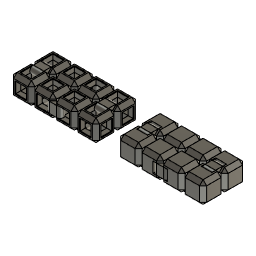
cubes v4 (Autodesk Fusion 360 design; units mm, degrees)
Autodesk Fusion 360 part; units mm, degrees
note: some values were not read from the file. Chosen so that the rebuilt part matches the saved one: which bodies a step acts on; which face or edge a step refers to. Set by a fixed rule: which sketch regions a step uses.
(part 1 of 2)
sketch "Sketch1" plane through (0, 0, 0) normal (0, 0, 1) x (1, 0, 0) in component "Cube"
  line L0 (0, 0) -> (50, 0)
  line L1 (50, 0) -> (50, -50)
  line L2 (50, -50) -> (0, -50)
  line L3 (0, -50) -> (0, 0)
  line L4 (50.2, 0) -> (100.2, 0)
  line L5 (100.2, 0) -> (100.2, -50)
  line L6 (100.2, -50) -> (50.2, -50)
  line L7 (50.2, -50) -> (50.2, 0)
  dimension "d1" = 50
  dimension "d2" = 50
  dimension "d3" = 50
  dimension "d4" = 50
  dimension "d5" = 0.2
  constraint horizontal L0
  constraint vertical L1
  constraint horizontal L2
  constraint vertical L3
  constraint coincident L0.start L3.end
  constraint horizontal L4
  constraint vertical L5
  constraint horizontal L6
  constraint vertical L7
  constraint collinear L0 L4
  measures "d1" distance of L1.end L2.end
  measures "d2" distance of L0.end L1.end
  measures "d3" distance of L4.start L4.end
  measures "d4" distance of L4.start L6.end
  measures "d5" distance of L1 L7
extrude "Extrude1" add sketch "Sketch1" along normal blind 50 makes body 1 at (16.6667, 0, 16.6667) makes body 2 at (100.2, -16.6667, 16.6667) in component "Cube"
sketch "Sketch2" plane through (0, 0, 0) normal (0, 0, -1) x (1, 0, 0) in component "Cube"
  line L0 (50, 50) -> (0, 50)
  line L1 (0, 50) -> (0, 0)
  line L2 (0, 0) -> (50, 0)
  line L3 (50, 0) -> (50, 50)
  line L4 (50, 12.5) -> (33.2333, 12.5)
  line L5 (33.2333, 12.5) -> (33.2333, 37.5)
  line L6 (33.2333, 37.5) -> (50, 37.5)
  line L7 (50, 37.5) -> (50, 12.5)
  line L8 (50.1, 12.7) -> (33.4333, 12.7)
  line L9 (33.4333, 12.7) -> (33.4333, 37.3)
  line L10 (33.4333, 37.3) -> (50.1, 37.3)
  line L11 (50.1, 37.3) -> (50.1, 12.7)
  line L12 (0, 25) -> (50, 25) construction
  dimension "d8" = 0.1
  dimension "d9" = 0.2
  dimension "d10" = 0.2
  dimension "d11" = 0.2
  dimension "d12" = 25
  dimension "d13" = 16.7667
  constraint horizontal L4
  constraint vertical L5
  constraint horizontal L6
  constraint vertical L7
  constraint coincident L3 L4.start
  constraint horizontal L8
  constraint vertical L9
  constraint horizontal L10
  constraint vertical L11
  constraint midpoint L1 L12.start
  constraint midpoint L3 L12.end
  constraint symmetric L4 L6 L12
  measures "d8" distance of L7 L11
  measures "d9" distance of L4 L8
  measures "d10" distance of L6 L10
  measures "d11" distance of L5 L9
  measures "d12" distance of L4.end L5.end
  measures "d13" distance of L4.start L4.end
sketch "Sketch3" plane through (0, 0, 0) normal (0, 0, -1) x (1, 0, 0) in component "Cube"
  line L0 (100.2, 50) -> (50.2, 50)
  line L1 (50.2, 50) -> (50.2, 0)
  line L2 (50.2, 0) -> (100.2, 0)
  line L3 (100.2, 0) -> (100.2, 50)
  line L4 (100.2, 25) -> (50.2, 25) construction
  line L5 (66.9667, 12.5) -> (50.2, 12.5)
  line L6 (50.2, 12.5) -> (50.2, 37.5)
  line L7 (50.2, 37.5) -> (66.9667, 37.5)
  line L8 (66.9667, 37.5) -> (66.9667, 12.5)
  line L9 (66.7667, 12.7) -> (50.1, 12.7)
  line L10 (50.1, 12.7) -> (50.1, 37.3)
  line L11 (50.1, 37.3) -> (66.7667, 37.3)
  line L12 (66.7667, 37.3) -> (66.7667, 12.7)
  dimension "d19" = 0.2
  dimension "d20" = 0.2
  dimension "d21" = 0.2
  dimension "d22" = 25
  dimension "d23" = 0.1
  dimension "d24" = 16.7667
  constraint midpoint L3 L4.start
  constraint midpoint L1 L4.end
  constraint horizontal L5
  constraint vertical L6
  constraint horizontal L7
  constraint vertical L8
  constraint coincident L1 L6.end
  constraint horizontal L9
  constraint vertical L10
  constraint horizontal L11
  constraint vertical L12
  constraint symmetric L4 L5 L7
  measures "d19" distance of L5 L9
  measures "d20" distance of L8 L12
  measures "d21" distance of L7 L11
  measures "d22" distance of L5.start L7.end
  measures "d23" distance of L6 L10
  measures "d24" distance of L5.start L5.end
sketch "Sketch4" plane through (0, 0, 50) normal (0, 0, 1) x (-1, 0, 0) in component "Cube"
  line L0 (0, 50) -> (-50, 50)
  line L1 (-50, 50) -> (-50, 0)
  line L2 (-50, 0) -> (0, 0)
  line L3 (0, 0) -> (0, 50)
  line L4 (-25, 50) -> (-25, 0) construction
  line L5 (-37.5, 16.7667) -> (-12.5, 16.7667)
  line L6 (-12.5, 16.7667) -> (-12.5, 0)
  line L7 (-12.5, 0) -> (-37.5, 0)
  line L8 (-37.5, 0) -> (-37.5, 16.7667)
  line L9 (-37.3, 16.5667) -> (-12.7, 16.5667)
  line L10 (-12.7, 16.5667) -> (-12.7, -0.1)
  line L11 (-12.7, -0.1) -> (-37.3, -0.1)
  line L12 (-37.3, -0.1) -> (-37.3, 16.5667)
  dimension "d25" = 0.1
  dimension "d26" = 0.2
  dimension "d27" = 0.2
  dimension "d28" = 25
  dimension "d29" = 0.2
  dimension "d30" = 16.7667
  constraint midpoint L0 L4.start
  constraint midpoint L2 L4.end
  constraint horizontal L5
  constraint vertical L6
  constraint horizontal L7
  constraint vertical L8
  constraint coincident L2 L6.end
  constraint horizontal L9
  constraint vertical L10
  constraint horizontal L11
  constraint vertical L12
  constraint symmetric L4 L6 L8
  measures "d25" distance of L7 L11
  measures "d26" distance of L8 L12
  measures "d27" distance of L6 L10
  measures "d28" distance of L5.start L5.end
  measures "d29" distance of L5 L9
  measures "d30" distance of L5.start L7.end
sketch "Sketch5" plane through (0, -50, 0) normal (0, -1, 0) x (1, 0, 0) in component "Cube"
  line L0 (50.2, 0) -> (100.2, 0)
  line L1 (100.2, 0) -> (100.2, 50)
  line L2 (100.2, 50) -> (50.2, 50)
  line L3 (50.2, 50) -> (50.2, 0)
  line L4 (100.2, 25) -> (50.2, 25) construction
  line L5 (100.2, 37.5) -> (83.4333, 37.5)
  line L6 (83.4333, 37.5) -> (83.4333, 12.5)
  line L7 (83.4333, 12.5) -> (100.2, 12.5)
  line L8 (100.2, 12.5) -> (100.2, 37.5)
  line L9 (100.3, 37.3) -> (83.6333, 37.3)
  line L10 (83.6333, 37.3) -> (83.6333, 12.7)
  line L11 (83.6333, 12.7) -> (100.3, 12.7)
  line L12 (100.3, 12.7) -> (100.3, 37.3)
  dimension "d87" = 16.7667
  dimension "d88" = 0.2
  dimension "d89" = 0.2
  dimension "d90" = 0.2
  dimension "d91" = 25
  dimension "d92" = 0.1
  constraint midpoint L1 L4.start
  constraint midpoint L3 L4.end
  constraint horizontal L5
  constraint vertical L6
  constraint horizontal L7
  constraint vertical L8
  constraint coincident L1 L5.start
  constraint horizontal L9
  constraint vertical L10
  constraint horizontal L11
  constraint vertical L12
  constraint symmetric L4 L5 L7
  measures "d87" distance of L5.start L5.end
  measures "d88" distance of L6 L10
  measures "d89" distance of L5 L9
  measures "d90" distance of L7 L11
  measures "d91" distance of L5.end L6.end
  measures "d92" distance of L8 L12
chamfer "Chamfer1" distance 8.3333 angle 45 24 edges at (0, 0, 25) (50, 0, 25) (25, 0, 0) (25, 0, 50) (50, -50, 25) (50, -25, 0) (50, -25, 50) (0, -50, 25) (25, -50, 0) (25, -50, 50) (0, -25, 0) (0, -25, 50) (50.2, 0, 25) (100.2, 0, 25) (75.2, 0, 0) (75.2, 0, 50) (100.2, -50, 25) (100.2, -25, 0) (100.2, -25, 50) (50.2, -50, 25) (75.2, -50, 0) (75.2, -50, 50) (50.2, -25, 0) (50.2, -25, 50) on bodies 1 2 in component "Cube"
extrude "Extrude2" cut sketch "Sketch2" sketch "Sketch3" against normal blind 16.8667 contours L3 L4 L5 L6 L7 L8 L9 L10 | L3 L7 L8 L9 L10 of sketch 2 contours L1 L5 L6 L7 L8 L9 L11 L12 | L1 L6 L9 L11 L12 bodies 1 2 in component "Cube"
extrude "Extrude3" add sketch "Sketch2" sketch "Sketch3" against normal blind 16.6667 separate body contours L3 L7 L8 L10 L11 | L3 L7 L8 L9 L10 of sketch 2 contours L1 L6 L9 L11 L12 | L1 L6 L9 L10 L11 makes body 3 in component "Cube"
fillet "Fillet1" radius 8.3333 4 edges at (33.4333, -25, 0) (33.4333, -25, 16.6667) (66.7667, -25, 0) (66.7667, -25, 16.6667) on bodies 3 in component "Cube"
extrude "Extrude4" cut sketch "Sketch5" against normal blind 16.8667 contours L1 L5 L6 L7 L8 L9 L10 L11 | L1 L8 L9 L10 L11 bodies 2 in component "Cube"
extrude "Extrude5" cut sketch "Sketch4" against normal blind 16.8667 contours L2 L5 L6 L7 L8 L9 L10 L12 | L2 L7 L9 L10 L12 bodies 1 in component "Cube"
extrude "Extrude6" add sketch "Sketch5" against normal blind 16.6667 separate body contours L1 L8 L9 L10 L11 | L1 L8 L9 L11 L12 makes body 4 in component "Cube"
extrude "Extrude7" add sketch "Sketch4" against normal blind 16.6667 separate body contours L2 L7 L10 L11 L12 | L2 L7 L9 L10 L12 makes body 5 in component "Cube"
fillet "Fillet2" radius 8.3333 2 edges at (25, -16.5667, 50) (25, -16.5667, 33.3333) on bodies 5 in component "Cube"
fillet "Fillet3" radius 8.3333 2 edges at (83.6333, -50, 25) (83.6333, -33.3333, 25) on bodies 4 in component "Cube"
sketch "Sketch6" plane through (0, 0, 12.7) normal (0, 0, -1) x (1, 0, 0) in component "Cube"
  arc A0 (91.9667, 50) -> (91.9667, 33.3333) centre (91.9667, 41.6667) ccw
  line L0 (91.9667, 33.3333) -> (100.3, 33.3333)
  line L1 (100.3, 33.3333) -> (100.3, 50)
  line L2 (100.3, 50) -> (91.9667, 50)
  circle A1 centre (91.9667, 41.6667) radius 4.1667
  circle A2 centre (91.9667, 41.6667) radius 4.4667
  dimension "d95" = 8.3333
  dimension "d102" = 0.3
  constraint concentric A0 A1
  measures "d95" diameter of A1
ref_plane "WorkPlane1" through (91.9667, -41.6667, 16.9667) normal (0, 0, -1) x (-1, 0, 0) in component "Cube"
sketch "Sketch7" plane through (36.55, -16.25, 16.9667) normal (0, 0, -1) x (-1, 0, 0) in component "Cube"
  circle A0 centre (-55.4167, -25.4167) radius 4.1667
  circle A1 centre (-55.4167, -25.4167) radius 4.3667
  dimension "d101" = 0.2
loft "Loft1" cut profiles "Sketch6" section 1 contours A1 | A2 section 2 point at (91.9667, -41.6667, 16.9667) bodies 4 in component "Cube"
sketch "Sketch10" plane through (0, 0, 12.5) normal (0, 0, 1) x (-1, 0, 0) in component "Cube"
  circle A0 centre (-91.9667, 41.6667) radius 4.1667
  circle A1 centre (-91.9667, 41.6667) radius 4.1667
  dimension "d103" = 8.3333
  constraint concentric A0 A1
  measures "d103" diameter of A1
ref_plane "WorkPlane3" through (91.8167, -41.5667, 16.6667) normal (0, 0, 1) x (1, 0, 0) in component "Cube"
sketch "Sketch11" plane through (36.4, -16.15, 16.6667) normal (0, 0, 1) x (-1, 0, 0) in component "Cube"
  point P0 (-55.5667, 25.5167)
loft "Loft3" add profiles "Sketch10" section 1 section 2 point at (91.9667, -41.6667, 16.6667) bodies 2 in component "Cube"
ref_plane "WorkPlane11" through (75.2, -50, 25) normal (0, 0, 1) x (-1, 0, 0) in component "Cube"
sketch "Sketch22" plane through (0, 0, 37.3) normal (0, 0, 1) x (-1, 0, 0) in component "Cube"
  arc A0 (-91.9667, 33.3333) -> (-91.9667, 50) centre (-91.9667, 41.6667) ccw
  line L0 (-91.9667, 50) -> (-100.3, 50)
  line L1 (-100.3, 50) -> (-100.3, 33.3333)
  line L2 (-100.3, 33.3333) -> (-91.9667, 33.3333)
  circle A1 centre (-91.9667, 41.6667) radius 4.1667
  dimension "d104" = 8.3333
  constraint concentric A0 A1
  measures "d104" diameter of A1
ref_plane "WorkPlane12" through (91.9667, -41.6667, 41.4667) normal (0, 0, 1) x (-1, 0, 0) in component "Cube"
sketch "Sketch23" plane through (45.3, -20, 41.4667) normal (0, 0, 1) x (1, 0, 0) in component "Cube"
  point P0 (46.6667, -21.6667)
loft "Loft12" add profiles "Sketch22" section 1 contours A1 section 2 point at (91.9667, -41.6667, 41.4667) bodies 4 in component "Cube"
sketch "Sketch24" plane through (0, 0, 37.5) normal (0, 0, -1) x (1, 0, 0) in component "Cube"
  line L0 (83.4333, 50) -> (83.4333, 33.1333)
  line L1 (83.4333, 33.1333) -> (100.2, 33.1333)
  circle A0 centre (91.9667, 41.6667) radius 4.3167
  line L2 (100.2, 41.6667) -> (91.8667, 50)
  line L3 (91.8667, 50) -> (83.4333, 50)
  line L4 (100.2, 33.1333) -> (100.2, 41.6667)
  point P0 (91.9667, 41.6667)
  dimension "d106" = 8.6333
  constraint coincident P0 A0.centre
  measures "d106" diameter of A0
ref_plane "WorkPlane13" through (91.8167, -41.5667, 41.7667) normal (0, 0, -1) x (1, 0, 0) in component "Cube"
sketch "Sketch26" plane through (45.15, -19.9, 41.7667) normal (0, 0, -1) x (1, 0, 0) in component "Cube"
  point P0 (46.8167, 21.7667)
loft "Loft13" cut profiles "Sketch24" section 1 contours A0 section 2 point at (91.9667, -41.6667, 41.7667) bodies 2 in component "Cube"
sketch "Sketch25" plane through (45.15, -19.9, 41.7667) normal (0, 0, -1) x (1, 0, 0) in component "Cube"
  point P0 (46.8167, 21.7667)
ref_plane "WorkPlane4" through (25, -25, 0) normal (0, -1, 0) x (1, 0, 0) in component "Cube"
ref_plane "WorkPlane5" through (25, -25, 50) normal (1, 0, 0) x (0, 1, 0) in component "Cube"
sketch "Sketch12" plane through (12.7, 0, 0) normal (-1, 0, 0) x (0, -1, 0) in component "Cube"
  arc A0 (8.2333, 33.3333) -> (8.2333, 50) centre (8.2333, 41.6667) ccw
  line L0 (8.2333, 50) -> (-0.1, 50)
  line L1 (-0.1, 50) -> (-0.1, 33.3333)
  line L2 (-0.1, 33.3333) -> (8.2333, 33.3333)
  circle A1 centre (8.2333, 41.6667) radius 4.1667
  dimension "d66" = 8.3333
  constraint concentric A0 A1
  measures "d66" diameter of A1
ref_plane "WorkPlane6" through (8.5333, -8.2333, 41.6667) normal (-1, 0, 0) x (0, -1, 0) in component "Cube"
sketch "Sketch13" plane through (8.5333, -3.55, 16.25) normal (-1, 0, 0) x (0, 1, 0) in component "Cube"
  point P0 (-4.6833, -25.4167)
loft "Loft4" add profiles "Sketch12" section 1 contours A1 section 2 point at (8.5333, -8.2333, 41.6667) bodies 5 in component "Cube"
sketch "Sketch14" plane through (12.5, 0, 0) normal (1, 0, 0) x (0, 1, 0) in component "Cube"
  line L0 (-16.7667, 50) -> (-16.7667, 33.1333)
  line L1 (-16.7667, 33.1333) -> (0, 33.1333)
  circle A0 centre (-8.2333, 41.6667) radius 4.3167
  circle A1 centre (-8.2333, 41.6667) radius 4.1667
  line L2 (0, 41.6667) -> (-8.3333, 50)
  line L3 (-8.3333, 50) -> (-16.7667, 50)
  line L4 (0, 33.1333) -> (0, 41.6667)
  dimension "d108" = 8.6333
  constraint concentric A0 A1
  measures "d108" diameter of A0
ref_plane "WorkPlane7" through (8.4333, -8.3833, 41.5667) normal (1, 0, 0) x (0, 1, 0) in component "Cube"
sketch "Sketch15" plane through (8.4333, -3.85, 16.05) normal (1, 0, 0) x (0, 1, 0) in component "Cube"
  point P0 (-4.3833, 25.6167)
loft "Loft5" cut profiles "Sketch14" section 1 contours A0 | A1 section 2 point at (8.4333, -8.2333, 41.6667) bodies 1 in component "Cube"
mirror "Mirror2" about plane through (25, -25, 50) normal (1, 0, 0) of "Loft4", "Loft5" in component "Cube"
sketch "Sketch16" plane through (0, -12.7, 0) normal (0, 1, 0) x (-1, 0, 0) in component "Cube"
  arc A0 (-58.4333, 16.6667) -> (-58.4333, 0) centre (-58.4333, 8.3333) ccw
  line L0 (-58.4333, 0) -> (-41.7667, 0)
  arc A1 (-41.7667, 0) -> (-41.7667, 16.6667) centre (-41.7667, 8.3333) ccw
  line L1 (-41.7667, 16.6667) -> (-58.4333, 16.6667)
  circle A2 centre (-58.4333, 8.3333) radius 4.1667
  circle A3 centre (-41.7667, 8.3333) radius 4.1667
  dimension "d72" = 8.3333
  dimension "d73" = 8.3333
  constraint concentric A0 A2
  constraint concentric A1 A3
  measures "d72" diameter of A2
  measures "d73" diameter of A3
ref_plane "WorkPlane8" through (50.1, -8.5333, 8.3333) normal (0, 1, 0) x (-1, 0, 0) in component "Cube"
sketch "Sketch17" plane through (20.2, -8.5333, 3.75) normal (0, 1, 0) x (1, 0, 0) in component "Cube"
  point P0 (38.2333, -4.5833)
  point P1 (21.5667, -4.5833)
loft "Loft6" add profiles "Sketch16" section 1 contours A2 section 2 point at (58.4333, -8.5333, 8.3333) bodies 3 in component "Cube"
loft "Loft7" add profiles "Sketch16" section 1 contours A3 section 2 point at (41.7667, -8.5333, 8.3333) bodies 3 in component "Cube"
sketch "Sketch18" plane through (0, -12.5, 0) normal (0, -1, 0) x (1, 0, 0) in component "Cube"
  line L0 (50, 16.8667) -> (33.2333, 16.8667)
  line L1 (33.2333, 16.8667) -> (33.2333, 0)
  circle A0 centre (41.7667, 8.3333) radius 4.1667
  circle A1 centre (41.7667, 8.3333) radius 4.4667
  line L2 (41.6667, 0) -> (50, 8.3333)
  line L3 (50, 8.3333) -> (50, 16.8667)
  line L4 (33.2333, 0) -> (41.6667, 0)
  dimension "d75" = 0.3
ref_plane "WorkPlane9" through (41.6167, -8.2333, 8.4333) normal (0, -1, 0) x (1, 0, 0) in component "Cube"
sketch "Sketch19" plane through (16.15, -8.2333, 3.95) normal (0, -1, 0) x (1, 0, 0) in component "Cube"
  point P0 (25.6167, 4.3833)
loft "Loft8" cut profiles "Sketch18" section 1 contours A0 | A1 section 2 point at (41.7667, -8.2333, 8.3333) bodies 1 in component "Cube"
sketch "Sketch20" plane through (0, -12.5, 0) normal (0, -1, 0) x (1, 0, 0) in component "Cube"
  line L0 (66.9667, 0) -> (66.9667, 16.8667)
  line L1 (66.9667, 16.8667) -> (50.2, 16.8667)
  circle A0 centre (58.4333, 8.3333) radius 4.1667
  circle A1 centre (58.4333, 8.3333) radius 4.4667
  line L2 (50.2, 8.3333) -> (58.5333, 0)
  line L3 (58.5333, 0) -> (66.9667, 0)
  line L4 (50.2, 16.8667) -> (50.2, 8.3333)
  point P0 (58.4333, 8.3333)
  dimension "d77" = 0.3
ref_plane "WorkPlane10" through (58.5833, -8.2333, 8.4333) normal (0, -1, 0) x (1, 0, 0) in component "Cube"
sketch "Sketch21" plane through (24.25, -8.2333, 3.95) normal (0, -1, 0) x (1, 0, 0) in component "Cube"
  point P0 (34.1833, 4.3833)
loft "Loft9" cut profiles "Sketch20" section 1 contours A0 | A1 section 2 point at (58.4333, -8.2333, 8.3333) bodies 2 in component "Cube"
mirror "Mirror3" about plane through (25, -25, 0) normal (0, -1, 0) of 4 faces at (40.4068, -11.7889, 11.7983) (57.0735, -11.7889, 4.8684) (60.5982, -12.0056, 5.6186) (40.0306, -12.0056, 11.3404) on bodies 1 2 3 in component "Cube"
mirror "Mirror4" about plane through (100.3, -50, 12.7) normal (1, 0, 0) of bodies 4 3 5 1 2 makes body 6 at (200.6, -30.5556, 30.5556) makes body 7 at (119.8444, -19.4444, 50) makes body 8 at (153.2783, -29.1, 0) makes body 9 at (100.3, -38.8889, 29.1) makes body 10 at (179.7, 0.1, 38.8889) in component "Cube"
combine "Combine2" operation add target body 4 tool bodies 9 in component "Cube"
mirror "Mirror5" about plane through (187.9, 0.1, 50) normal (0, 1, 0) of bodies 10 4 2 8 1 5 7 3 6 makes body 11 at (0, 30.7556, 30.5556) makes body 12 at (80.7556, 30.7556, 50) makes body 13 at (52.8783, 21.1, 0) makes body 14 at (97.5217, 50.2, 29.1) makes body 15 at (20.9, 0.1, 38.8889) makes body 16 at (200.6, 30.7556, 30.5556) makes body 17 at (119.8444, 19.6444, 50) makes body 18 at (147.7217, 29.3, 0) makes body 19 at (179.7, 0.1, 38.8889) in component "Cube"
combine "Combine3" operation add target body 5 tool bodies 15 in component "Cube"
combine "Combine4" operation add target body 10 tool bodies 19 in component "Cube"
sketch "Sketch1 (2)" plane through (0, 0, 0) normal (0, 0, 1) x (1, 0, 0) in component "Holey Cube"
  line L0 (0, 0) -> (50, 0)
  line L1 (50, 0) -> (50, -50)
  line L2 (50, -50) -> (0, -50)
  line L3 (0, -50) -> (0, 0)
  line L4 (50.2, 0) -> (100.2, 0)
  line L5 (100.2, 0) -> (100.2, -50)
  line L6 (100.2, -50) -> (50.2, -50)
  line L7 (50.2, -50) -> (50.2, 0)
  dimension "d1_4" = 50
  dimension "d2_4" = 50
  dimension "d3_4" = 50
  dimension "d4_4" = 50
  dimension "d5_4" = 0.2
  constraint horizontal L0
  constraint vertical L1
  constraint horizontal L2
  constraint vertical L3
  constraint coincident L0.start L3.end
  constraint horizontal L4
  constraint vertical L5
  constraint horizontal L6
  constraint vertical L7
  constraint collinear L0 L4
  measures "d1_4" distance of L1.end L2.end
  measures "d2_4" distance of L0.end L1.end
  measures "d3_4" distance of L4.start L4.end
  measures "d4_4" distance of L4.start L6.end
  measures "d5_4" distance of L1 L7
extrude "Extrude1'" add sketch "Sketch1 (2)" along normal blind 50 separate body makes body 20 at (16.6667, 0, 16.6667) makes body 21 at (100.2, -16.6667, 16.6667) in component "Holey Cube"
sketch "Sketch2 (2)" plane through (0, 0, 0) normal (0, 0, -1) x (1, 0, 0) in component "Holey Cube"
  line L0 (50, 50) -> (0, 50)
  line L1 (0, 50) -> (0, 0)
  line L2 (0, 0) -> (50, 0)
  line L3 (50, 0) -> (50, 50)
  line L4 (50, 12.5) -> (33.2333, 12.5)
  line L5 (33.2333, 12.5) -> (33.2333, 37.5)
  line L6 (33.2333, 37.5) -> (50, 37.5)
  line L7 (50, 37.5) -> (50, 12.5)
  line L8 (50.1, 12.7) -> (33.4333, 12.7)
  line L9 (33.4333, 12.7) -> (33.4333, 37.3)
  line L10 (33.4333, 37.3) -> (50.1, 37.3)
  line L11 (50.1, 37.3) -> (50.1, 12.7)
  line L12 (0, 25) -> (50, 25) construction
  dimension "d8_4" = 0.1
  dimension "d9_4" = 0.2
  dimension "d10_4" = 0.2
  dimension "d11_4" = 0.2
  dimension "d12_4" = 25
  dimension "d13_4" = 16.7667
  constraint horizontal L4
  constraint vertical L5
  constraint horizontal L6
  constraint vertical L7
  constraint coincident L3 L4.start
  constraint horizontal L8
  constraint vertical L9
  constraint horizontal L10
  constraint vertical L11
  constraint midpoint L1 L12.start
  constraint midpoint L3 L12.end
  constraint symmetric L4 L6 L12
  measures "d8_4" distance of L7 L11
  measures "d9_4" distance of L4 L8
  measures "d10_4" distance of L6 L10
  measures "d11_4" distance of L5 L9
  measures "d12_4" distance of L4.end L5.end
  measures "d13_4" distance of L4.start L4.end
sketch "Sketch3 (2)" plane through (0, 0, 0) normal (0, 0, -1) x (1, 0, 0) in component "Holey Cube"
  line L0 (100.2, 50) -> (50.2, 50)
  line L1 (50.2, 50) -> (50.2, 0)
  line L2 (50.2, 0) -> (100.2, 0)
  line L3 (100.2, 0) -> (100.2, 50)
  line L4 (100.2, 25) -> (50.2, 25) construction
  line L5 (66.9667, 12.5) -> (50.2, 12.5)
  line L6 (50.2, 12.5) -> (50.2, 37.5)
  line L7 (50.2, 37.5) -> (66.9667, 37.5)
  line L8 (66.9667, 37.5) -> (66.9667, 12.5)
  line L9 (66.7667, 12.7) -> (50.1, 12.7)
  line L10 (50.1, 12.7) -> (50.1, 37.3)
  line L11 (50.1, 37.3) -> (66.7667, 37.3)
  line L12 (66.7667, 37.3) -> (66.7667, 12.7)
  dimension "d19_4" = 0.2
  dimension "d20_4" = 0.2
  dimension "d21_4" = 0.2
  dimension "d22_4" = 25
  dimension "d23_4" = 0.1
  dimension "d24_4" = 16.7667
  constraint midpoint L3 L4.start
  constraint midpoint L1 L4.end
  constraint horizontal L5
  constraint vertical L6
  constraint horizontal L7
  constraint vertical L8
  constraint coincident L1 L6.end
  constraint horizontal L9
  constraint vertical L10
  constraint horizontal L11
  constraint vertical L12
  constraint symmetric L4 L5 L7
  measures "d19_4" distance of L5 L9
  measures "d20_4" distance of L8 L12
  measures "d21_4" distance of L7 L11
  measures "d22_4" distance of L5.start L7.end
  measures "d23_4" distance of L6 L10
  measures "d24_4" distance of L5.start L5.end
sketch "Sketch4 (2)" plane through (0, 0, 50) normal (0, 0, 1) x (-1, 0, 0) in component "Holey Cube"
  line L0 (0, 50) -> (-50, 50)
  line L1 (-50, 50) -> (-50, 0)
  line L2 (-50, 0) -> (0, 0)
  line L3 (0, 0) -> (0, 50)
  line L4 (-25, 50) -> (-25, 0) construction
  line L5 (-37.5, 16.7667) -> (-12.5, 16.7667)
  line L6 (-12.5, 16.7667) -> (-12.5, 0)
  line L7 (-12.5, 0) -> (-37.5, 0)
  line L8 (-37.5, 0) -> (-37.5, 16.7667)
  line L9 (-37.3, 16.5667) -> (-12.7, 16.5667)
  line L10 (-12.7, 16.5667) -> (-12.7, -0.1)
  line L11 (-12.7, -0.1) -> (-37.3, -0.1)
  line L12 (-37.3, -0.1) -> (-37.3, 16.5667)
  line L13 (0, 25) -> (-50, 25) construction
  line L14 (-12.5, 12.5) -> (-37.5, 12.5)
  line L15 (-37.5, 12.5) -> (-37.5, 37.5)
  line L16 (-37.5, 37.5) -> (-12.5, 37.5)
  line L17 (-12.5, 37.5) -> (-12.5, 12.5)
  dimension "d25_4" = 0.1
  dimension "d26_4" = 0.2
  dimension "d27_4" = 0.2
  dimension "d28_4" = 25
  dimension "d29_4" = 0.2
  dimension "d30_4" = 16.7667
  dimension "d166" = 25
  dimension "d167" = 25
  constraint midpoint L0 L4.start
  constraint midpoint L2 L4.end
  constraint horizontal L5
  constraint vertical L6
  constraint horizontal L7
  constraint vertical L8
  constraint coincident L2 L6.end
  constraint horizontal L9
  constraint vertical L10
  constraint horizontal L11
  constraint vertical L12
  constraint symmetric L4 L6 L8
  constraint midpoint L3 L13.start
  constraint midpoint L1 L13.end
  constraint horizontal L14
  constraint vertical L15
  constraint horizontal L16
  constraint vertical L17
  constraint symmetric L4 L15 L17
  constraint symmetric L13 L14 L16
  measures "d25_4" distance of L7 L11
  measures "d26_4" distance of L8 L12
  measures "d27_4" distance of L6 L10
  measures "d28_4" distance of L5.start L5.end
  measures "d29_4" distance of L5 L9
  measures "d30_4" distance of L5.start L7.end
  measures "d166" distance of L15.end L16.end
  measures "d167" distance of L14.start L16.end
extrude "Extrude11" cut sketch "Sketch4 (2)" against normal up to surface (50 mm away) contours L5 L6 L8 L9 L10 L12 L14 L15 L17 | L9 L10 L12 L14 | L5 L15 L16 L17 bodies 20 in component "Holey Cube"
sketch "Sketch5 (2)" plane through (0, -50, 0) normal (0, -1, 0) x (1, 0, 0) in component "Holey Cube"
  line L0 (135.5199, 25) -> (64.8801, 25) construction
  line L1 (100.2, 37.5) -> (83.4333, 37.5)
  line L2 (83.4333, 37.5) -> (83.4333, 12.5)
  line L3 (83.4333, 12.5) -> (100.2, 12.5)
  line L4 (100.2, 12.5) -> (100.2, 37.5)
  line L5 (100.3, 37.3) -> (83.6333, 37.3)
  line L6 (83.6333, 37.3) -> (83.6333, 12.7)
  line L7 (83.6333, 12.7) -> (100.3, 12.7)
  line L8 (100.3, 12.7) -> (100.3, 37.3)
  line L9 (75.2, 62.5) -> (75.2, 37.5) construction
  line L10 (62.7, 37.5) -> (87.7, 37.5)
  line L11 (87.7, 37.5) -> (87.7, 12.5)
  line L12 (87.7, 12.5) -> (62.7, 12.5)
  line L13 (62.7, 12.5) -> (62.7, 37.5)
  line L14 (50.2, 0) -> (100.2, 0)
  line L15 (100.2, 0) -> (100.2, 50)
  line L16 (100.2, 50) -> (50.2, 50)
  line L17 (50.2, 50) -> (50.2, 0)
  line L18 (100.2, 0) -> (100.2, 50)
  dimension "d87_2" = 16.7667
  dimension "d88_2" = 0.2
  dimension "d89_2" = 0.2
  dimension "d90_2" = 0.2
  dimension "d91_2" = 25
  dimension "d92_2" = 0.1
  dimension "d154" = 25
  dimension "d155" = 25
  constraint horizontal L1
  constraint vertical L2
  constraint horizontal L3
  constraint vertical L4
  constraint horizontal L5
  constraint vertical L6
  constraint horizontal L7
  constraint vertical L8
  constraint symmetric L0 L1 L3
  constraint horizontal L10
  constraint vertical L11
  constraint horizontal L12
  constraint vertical L13
  constraint symmetric L9 L11 L13
  constraint symmetric L0 L10 L12
  constraint collinear L4 L18
  constraint midpoint L0 L15
  constraint midpoint L9 L16
  measures "d87_2" distance of L1.start L1.end
  measures "d88_2" distance of L2 L6
  measures "d89_2" distance of L1 L5
  measures "d90_2" distance of L3 L7
  measures "d91_2" distance of L1.end L2.end
  measures "d92_2" distance of L4 L8
  measures "d154" distance of L10.start L12.end
  measures "d155" distance of L10.start L10.end
extrude "Extrude8" cut sketch "Sketch5 (2)" against normal up to surface (50 mm away) contours L1 L2 L3 L5 L6 L7 L10 L11 L12 | L2 L10 L12 L13 | L5 L6 L7 L11 bodies 21 in component "Holey Cube"
sketch "Sketch27" plane through (100.2, 0, 0) normal (1, 0, 0) x (0, 1, 0) in component "Holey Cube"
  line L0 (-25, 58.3333) -> (-25, 41.6667) construction
  line L1 (-58.3333, 25) -> (-41.6667, 25) construction
  line L2 (-37.5, 37.5) -> (-12.5, 37.5)
  line L3 (-12.5, 37.5) -> (-12.5, 12.5)
  line L4 (-12.5, 12.5) -> (-37.5, 12.5)
  line L5 (-37.5, 12.5) -> (-37.5, 37.5)
  line L6 (0, 0) -> (0, 50)
  line L7 (-50, 50) -> (-50, 0)
  line L8 (-50, 0) -> (0, 0)
  line L9 (0, 50) -> (-50, 50)
  dimension "d158" = 25
  dimension "d159" = 25
  constraint horizontal L2
  constraint vertical L3
  constraint horizontal L4
  constraint vertical L5
  constraint symmetric L0 L3 L5
  constraint symmetric L1 L2 L4
  constraint midpoint L0 L9
  constraint midpoint L1 L7
  measures "d158" distance of L2.start L2.end
  measures "d159" distance of L2.start L4.end
extrude "Extrude9" cut sketch "Sketch27" against normal up to surface (100.2 mm away) contours L2 L3 L4 L5 bodies 20 21 in component "Holey Cube"
sketch "Sketch28" plane through (0, -50, 0) normal (0, -1, 0) x (1, 0, 0) in component "Holey Cube"
  line L0 (25, 58.3333) -> (25, 41.6667) construction
  line L1 (-8.3333, 25) -> (8.3333, 25) construction
  line L2 (12.5, 37.5) -> (37.5, 37.5)
  line L3 (37.5, 37.5) -> (37.5, 12.5)
  line L4 (37.5, 12.5) -> (12.5, 12.5)
  line L5 (12.5, 12.5) -> (12.5, 37.5)
  line L6 (0, 0) -> (50, 0)
  line L7 (50, 0) -> (50, 50)
  line L8 (50, 50) -> (0, 50)
  line L9 (0, 50) -> (0, 0)
  dimension "d162" = 25
  dimension "d163" = 25
  constraint horizontal L2
  constraint vertical L3
  constraint horizontal L4
  constraint vertical L5
  constraint symmetric L0 L3 L5
  constraint symmetric L1 L2 L4
  constraint midpoint L1 L9
  constraint midpoint L0 L8
  measures "d162" distance of L2.start L2.end
  measures "d163" distance of L2.start L4.end
extrude "Extrude10" cut sketch "Sketch28" against normal up to surface (50 mm away) contours L2 L3 L4 L5 bodies 20 in component "Holey Cube"
sketch "Sketch29" plane through (0, 0, 50) normal (0, 0, 1) x (-1, 0, 0) in component "Holey Cube"
  line L0 (-50.2, 50) -> (-100.2, 50)
  line L1 (-100.2, 50) -> (-100.2, 0)
  line L2 (-100.2, 0) -> (-50.2, 0)
  line L3 (-50.2, 0) -> (-50.2, 50)
  line L4 (-75.2, 66.5287) -> (-75.2, 33.4713) construction
  line L5 (-112.1292, 25) -> (-88.2708, 25) construction
  line L6 (-87.7, 12.5) -> (-62.7, 12.5)
  line L7 (-62.7, 12.5) -> (-62.7, 37.5)
  line L8 (-62.7, 37.5) -> (-87.7, 37.5)
  line L9 (-87.7, 37.5) -> (-87.7, 12.5)
  point P0 (-75.2, 50)
  point P1 (-50, 25)
  dimension "d175" = 25
  dimension "d176" = 25
  constraint vertical L4
  constraint perpendicular L1 L5
  constraint midpoint L0 L4
  constraint midpoint L1 L5
  constraint horizontal L6
  constraint vertical L7
  constraint horizontal L8
  constraint vertical L9
  constraint symmetric L5 L6 L8
  constraint symmetric L4 L7 L9
  measures "d175" distance of L6.start L6.end
  measures "d176" distance of L6.end L7.end
extrude "Extrude12" cut sketch "Sketch29" against normal up to surface (50 mm away) contours L6 L7 L8 L9 bodies 21 in component "Holey Cube"
extrude "Extrude2'" cut sketch "Sketch2 (2)" sketch "Sketch3 (2)" against normal blind 16.8667 contours L3 L4 L5 L6 L7 L8 L9 L10 | L3 L7 L8 L9 L10 of sketch 2 contours L1 L5 L6 L7 L8 L9 L11 L12 | L1 L6 L9 L11 L12 bodies 20 21 in component "Holey Cube"
extrude "Extrude3'" add sketch "Sketch2 (2)" sketch "Sketch3 (2)" against normal blind 16.6667 separate body contours L3 L7 L8 L10 L11 | L3 L7 L8 L9 L10 of sketch 2 contours L1 L6 L9 L11 L12 | L1 L6 L9 L10 L11 makes body 22 in component "Holey Cube"
fillet "Fillet1'" radius 8.3333 4 edges at (33.4333, -25, 0) (33.4333, -25, 16.6667) (66.7667, -25, 0) (66.7667, -25, 16.6667) on bodies 22 in component "Holey Cube"
extrude "Extrude4'" cut sketch "Sketch5 (2)" against normal blind 16.8667 contours L1 L4 L5 L11 L15 L18 | L1 L2 L3 L5 L6 L7 L10 L11 L12 | L4 L5 L7 L11 L15 L18 | L5 L6 L7 L11 | L3 L4 L7 L11 L15 L18 bodies 21 in component "Holey Cube"
extrude "Extrude5'" cut sketch "Sketch4 (2)" against normal blind 16.8667 contours L2 L6 L7 L10 L14 | L2 L7 L8 L12 L14 | L2 L7 L10 L12 L14 | L5 L6 L8 L9 L10 L12 L14 L15 L17 | L9 L10 L12 L14 bodies 20 in component "Holey Cube"
extrude "Extrude6'" add sketch "Sketch5 (2)" against normal blind 16.6667 separate body contours L4 L5 L7 L8 L15 L18 | L4 L5 L7 L11 L15 L18 | L5 L6 L7 L11 makes body 23 in component "Holey Cube"
extrude "Extrude7'" add sketch "Sketch4 (2)" against normal blind 16.6667 separate body contours L2 L7 L10 L11 L12 | L2 L7 L10 L12 L14 | L9 L10 L12 L14 makes body 24 in component "Holey Cube"
fillet "Fillet2'" radius 8.3333 2 edges at (25, -16.5667, 50) (25, -16.5667, 33.3333) on bodies 24 in component "Holey Cube"
fillet "Fillet3'" radius 8.3333 2 edges at (83.6333, -50, 25) (83.6333, -33.3333, 25) on bodies 23 in component "Holey Cube"
chamfer "Chamfer1'" distance 8.3333 angle 45 28 edges at (6.25, 0, 50) (43.75, 0, 50) (0, 0, 25) (25, 0, 0) (50, 0, 25) (50, -25, 50) (25, -50, 50) (0, -25, 50) (0, -50, 25) (0, -25, 0) (50, -50, 25) (25, -50, 0) (50, -43.75, 0) (50, -6.25, 0) (50.2, 0, 25) (75.2, 0, 0) (100.2, 0, 25) (75.2, 0, 50) (100.2, -25, 50) (75.2, -50, 50) (50.2, -25, 50) (50.2, -50, 25) (75.2, -50, 0) (100.2, -50, 6.25) (100.2, -50, 43.75) (100.2, -25, 0) (50.2, -43.75, 0) (50.2, -6.25, 0) on bodies 20 21 in component "Holey Cube"
chamfer "Chamfer2" distance 1.0417 angle 45 47 edges at (25, -37.5, 50) (37.5, -22.9167, 50) (12.5, -22.9167, 50) (12.5, -4.1667, 45.8333) (12.5, 0, 27.0833) (25, 0, 12.5) (37.5, 0, 27.0833) (37.5, -4.1667, 45.8333) (0, -25, 37.5) (0, -12.5, 25) (0, -25, 12.5) (0, -37.5, 25) (25, -50, 37.5) (12.5, -50, 25) (25, -50, 12.5) (37.5, -50, 25) (27.0833, -12.5, 0) (12.5, -25, 0) (27.0833, -37.5, 0) (50, -12.5, 22.9167) (50, -25, 37.5) (50, -37.5, 22.9167) (45.8333, -37.5, 4.1667) (45.8333, -12.5, 4.1667) (87.7, 0, 25) (75.2, 0, 37.5) (62.7, 0, 25) (75.2, 0, 12.5) (96.0333, -45.8333, 37.5) (77.2833, -50, 37.5) (62.7, -50, 25) (77.2833, -50, 12.5) (96.0333, -45.8333, 12.5) (100.2, -27.0833, 37.5) (100.2, -12.5, 25) (100.2, -27.0833, 12.5) (73.1167, -37.5, 0) (73.1167, -12.5, 0) (54.3667, -37.5, 4.1667) (50.2, -37.5, 22.9167) (50.2, -25, 37.5) (50.2, -12.5, 22.9167) (54.3667, -12.5, 4.1667) (62.7, -25, 50) (75.2, -12.5, 50) (87.7, -25, 50) (75.2, -37.5, 50) on bodies 20 21 in component "Holey Cube"
sketch "Sketch6 (2)" plane through (0, 0, 12.7) normal (0, 0, -1) x (1, 0, 0) in component "Holey Cube"
  arc A0 (91.9667, 50) -> (91.9667, 33.3333) centre (91.9667, 41.6667) ccw
  line L0 (91.9667, 33.3333) -> (100.3, 33.3333)
  line L1 (100.3, 33.3333) -> (100.3, 50)
  line L2 (100.3, 50) -> (91.9667, 50)
  circle A1 centre (91.9667, 41.6667) radius 4.1667
  circle A2 centre (91.9667, 41.6667) radius 4.4667
  dimension "d95_2" = 8.3333
  dimension "d102_2" = 0.3
  constraint concentric A0 A1
  measures "d95_2" diameter of A1
ref_plane "WorkPlane1" through (91.9667, -41.6667, 16.9667) normal (0, 0, -1) x (-1, 0, 0) in component "Holey Cube"
sketch "Sketch7 (2)" plane through (36.55, -16.25, 16.9667) normal (0, 0, -1) x (-1, 0, 0) in component "Holey Cube"
  circle A0 centre (-55.4167, -25.4167) radius 4.1667
  circle A1 centre (-55.4167, -25.4167) radius 4.3667
  dimension "d101_1" = 0.2
loft "Loft1'" cut profiles "Sketch6 (2)" section 1 contours A1 | A2 section 2 point at (91.9667, -41.6667, 16.9667) bodies 23 in component "Holey Cube"
sketch "Sketch10 (2)" plane through (0, 0, 12.5) normal (0, 0, 1) x (-1, 0, 0) in component "Holey Cube"
  circle A0 centre (-91.9667, 41.6667) radius 4.1667
  circle A1 centre (-91.9667, 41.6667) radius 4.1667
  dimension "d103_1" = 8.3333
  constraint concentric A0 A1
  measures "d103_1" diameter of A1
ref_plane "WorkPlane3" through (81.45, -31.25, 16.6667) normal (0, 0, 1) x (1, 0, 0) in component "Holey Cube"
sketch "Sketch11 (2)" plane through (36.4, -16.15, 16.6667) normal (0, 0, 1) x (-1, 0, 0) in component "Holey Cube"
  point P0 (-55.5667, 25.5167)
loft "Loft3'" add profiles "Sketch10 (2)" section 1 section 2 point at (91.9667, -41.6667, 16.6667) bodies 21 in component "Holey Cube"
ref_plane "WorkPlane11" through (100.2, -50, 25) normal (0, 0, 1) x (-1, 0, 0) in component "Holey Cube"
sketch "Sketch22 (2)" plane through (0, 0, 37.3) normal (0, 0, 1) x (-1, 0, 0) in component "Holey Cube"
  arc A0 (-91.9667, 33.3333) -> (-91.9667, 50) centre (-91.9667, 41.6667) ccw
  line L0 (-91.9667, 50) -> (-100.3, 50)
  line L1 (-100.3, 50) -> (-100.3, 33.3333)
  line L2 (-100.3, 33.3333) -> (-91.9667, 33.3333)
  circle A1 centre (-91.9667, 41.6667) radius 4.1667
  dimension "d104_1" = 8.3333
  constraint concentric A0 A1
  measures "d104_1" diameter of A1
ref_plane "WorkPlane12" through (91.9667, -41.6667, 41.4667) normal (0, 0, 1) x (-1, 0, 0) in component "Holey Cube"
sketch "Sketch23 (2)" plane through (45.3, -20, 41.4667) normal (0, 0, 1) x (1, 0, 0) in component "Holey Cube"
  point P0 (46.6667, -21.6667)
loft "Loft12'" add profiles "Sketch22 (2)" section 1 contours A1 section 2 point at (91.9667, -41.6667, 41.4667) bodies 23 in component "Holey Cube"
sketch "Sketch24 (2)" plane through (0, 0, 37.5) normal (0, 0, -1) x (1, 0, 0) in component "Holey Cube"
  circle A0 centre (91.9667, 41.6667) radius 4.3167
  line L0 (87.7, 12.5) -> (99.1583, 12.5)
  line L1 (99.1583, 12.5) -> (99.1583, 41.2352)
  line L2 (99.1583, 41.2352) -> (91.4352, 48.9583)
  line L3 (91.4352, 48.9583) -> (62.7, 48.9583)
  line L4 (62.7, 48.9583) -> (62.7, 37.5)
  line L5 (62.7, 37.5) -> (87.7, 37.5)
  line L6 (87.7, 37.5) -> (87.7, 12.5)
  point P0 (91.9667, 41.6667)
  dimension "d106_1" = 8.6333
  constraint coincident P0 A0.centre
  measures "d106_1" diameter of A0
ref_plane "WorkPlane13" through (81.45, -31.25, 41.7667) normal (0, 0, -1) x (-1, 0, 0) in component "Holey Cube"
sketch "Sketch26 (2)" plane through (45.15, -19.9, 41.7667) normal (0, 0, -1) x (1, 0, 0) in component "Holey Cube"
  point P0 (46.8167, 21.7667)
loft "Loft13'" cut profiles "Sketch24 (2)" section 1 contours A0 section 2 point at (91.9667, -41.6667, 41.7667) bodies 21 in component "Holey Cube"
sketch "Sketch25 (2)" plane through (45.15, -19.9, 41.7667) normal (0, 0, -1) x (1, 0, 0) in component "Holey Cube"
  point P0 (46.8167, 21.7667)
ref_plane "WorkPlane4" through (25, -25, 0) normal (0, -1, 0) x (1, 0, 0) in component "Holey Cube"
ref_plane "WorkPlane5" through (25, -25, 50) normal (1, 0, 0) x (0, 1, 0) in component "Holey Cube"
sketch "Sketch12 (2)" plane through (12.7, 0, 0) normal (-1, 0, 0) x (0, -1, 0) in component "Holey Cube"
  arc A0 (8.2333, 33.3333) -> (8.2333, 50) centre (8.2333, 41.6667) ccw
  line L0 (8.2333, 50) -> (-0.1, 50)
  line L1 (-0.1, 50) -> (-0.1, 33.3333)
  line L2 (-0.1, 33.3333) -> (8.2333, 33.3333)
  circle A1 centre (8.2333, 41.6667) radius 4.1667
  dimension "d66_3" = 8.3333
  constraint concentric A0 A1
  measures "d66_3" diameter of A1
ref_plane "WorkPlane6" through (8.5333, -8.2333, 41.6667) normal (-1, 0, 0) x (0, -1, 0) in component "Holey Cube"
sketch "Sketch13 (2)" plane through (8.5333, -3.55, 16.25) normal (-1, 0, 0) x (0, 1, 0) in component "Holey Cube"
  point P0 (-4.6833, -25.4167)
loft "Loft4'" add profiles "Sketch12 (2)" section 1 contours A1 section 2 point at (8.5333, -8.2333, 41.6667) bodies 24 in component "Holey Cube"
sketch "Sketch14 (2)" plane through (12.5, 0, 0) normal (1, 0, 0) x (0, 1, 0) in component "Holey Cube"
  circle A0 centre (-8.2333, 41.6667) radius 4.3167
  circle A1 centre (-8.2333, 41.6667) radius 4.1667
  line L0 (-37.5, 48.9583) -> (-37.5, 37.5)
  line L1 (-37.5, 37.5) -> (-12.5, 37.5)
  line L2 (-12.5, 37.5) -> (-12.5, 12.5)
  line L3 (-1.0417, 12.5) -> (-1.0417, 41.2352)
  line L4 (-1.0417, 41.2352) -> (-8.7648, 48.9583)
  line L5 (-8.7648, 48.9583) -> (-37.5, 48.9583)
  line L6 (-12.5, 12.5) -> (-1.0417, 12.5)
  dimension "d108_2" = 8.6333
  constraint concentric A0 A1
  measures "d108_2" diameter of A0
ref_plane "WorkPlane7" through (8.4333, -18.75, 31.25) normal (1, 0, 0) x (0, -1, 0) in component "Holey Cube"
sketch "Sketch15 (2)" plane through (8.4333, -3.85, 16.05) normal (1, 0, 0) x (0, 1, 0) in component "Holey Cube"
  point P0 (-4.3833, 25.6167)
loft "Loft5'" cut profiles "Sketch14 (2)" section 1 contours A0 | A1 section 2 point at (8.4333, -8.2333, 41.6667) bodies 20 in component "Holey Cube"
mirror "Mirror2'" about plane through (25, -25, 50) normal (1, 0, 0) of "Loft4'", "Loft5'" in component "Holey Cube"
sketch "Sketch16 (2)" plane through (0, -12.7, 0) normal (0, 1, 0) x (-1, 0, 0) in component "Holey Cube"
  arc A0 (-58.4333, 16.6667) -> (-58.4333, 0) centre (-58.4333, 8.3333) ccw
  line L0 (-58.4333, 0) -> (-41.7667, 0)
  arc A1 (-41.7667, 0) -> (-41.7667, 16.6667) centre (-41.7667, 8.3333) ccw
  line L1 (-41.7667, 16.6667) -> (-58.4333, 16.6667)
  circle A2 centre (-58.4333, 8.3333) radius 4.1667
  circle A3 centre (-41.7667, 8.3333) radius 4.1667
  dimension "d72_4" = 8.3333
  dimension "d73_4" = 8.3333
  constraint concentric A0 A2
  constraint concentric A1 A3
  measures "d72_4" diameter of A2
  measures "d73_4" diameter of A3
ref_plane "WorkPlane8" through (50.1, -8.5333, 8.3333) normal (0, 1, 0) x (-1, 0, 0) in component "Holey Cube"
sketch "Sketch17 (2)" plane through (20.2, -8.5333, 3.75) normal (0, 1, 0) x (1, 0, 0) in component "Holey Cube"
  point P0 (38.2333, -4.5833)
  point P1 (21.5667, -4.5833)
loft "Loft6'" add profiles "Sketch16 (2)" section 1 contours A2 section 2 point at (58.4333, -8.5333, 8.3333) bodies 22 in component "Holey Cube"
loft "Loft7'" add profiles "Sketch16 (2)" section 1 contours A3 section 2 point at (41.7667, -8.5333, 8.3333) bodies 22 in component "Holey Cube"
sketch "Sketch18 (2)" plane through (0, -12.5, 0) normal (0, -1, 0) x (1, 0, 0) in component "Holey Cube"
  circle A0 centre (41.7667, 8.3333) radius 4.1667
  circle A1 centre (41.7667, 8.3333) radius 4.4667
  line L0 (37.5, 12.5) -> (12.5, 12.5)
  line L1 (12.5, 12.5) -> (12.5, 1.0417)
  line L2 (48.9583, 8.7648) -> (48.9583, 37.5)
  line L3 (48.9583, 37.5) -> (37.5, 37.5)
  line L4 (37.5, 37.5) -> (37.5, 12.5)
  line L5 (12.5, 1.0417) -> (41.2352, 1.0417)
  line L6 (41.2352, 1.0417) -> (48.9583, 8.7648)
  dimension "d75_3" = 0.3
ref_plane "WorkPlane9" through (31.25, -8.2333, 18.75) normal (0, -1, 0) x (-1, 0, 0) in component "Holey Cube"
sketch "Sketch19 (2)" plane through (16.15, -8.2333, 3.95) normal (0, -1, 0) x (1, 0, 0) in component "Holey Cube"
  point P0 (25.6167, 4.3833)
loft "Loft8'" cut profiles "Sketch18 (2)" section 1 contours A0 | A1 section 2 point at (41.7667, -8.2333, 8.3333) bodies 20 in component "Holey Cube"
sketch "Sketch20 (2)" plane through (0, -12.5, 0) normal (0, -1, 0) x (1, 0, 0) in component "Holey Cube"
  circle A0 centre (58.4333, 8.3333) radius 4.1667
  circle A1 centre (58.4333, 8.3333) radius 4.4667
  line L0 (62.7, 12.5) -> (62.7, 37.5)
  line L1 (62.7, 37.5) -> (51.2417, 37.5)
  line L2 (87.7, 12.5) -> (62.7, 12.5)
  line L3 (58.9648, 1.0417) -> (87.7, 1.0417)
  line L4 (51.2417, 37.5) -> (51.2417, 8.7648)
  line L5 (51.2417, 8.7648) -> (58.9648, 1.0417)
  line L6 (87.7, 1.0417) -> (87.7, 12.5)
  point P0 (58.4333, 8.3333)
  dimension "d77_3" = 0.3
ref_plane "WorkPlane10" through (31.25, -8.2333, 18.75) normal (0, -1, 0) x (-1, 0, 0) in component "Holey Cube"
sketch "Sketch21 (2)" plane through (24.25, -8.2333, 3.95) normal (0, -1, 0) x (1, 0, 0) in component "Holey Cube"
  point P0 (34.1833, 4.3833)
loft "Loft9'" cut profiles "Sketch20 (2)" section 1 contours A0 | A1 section 2 point at (58.4333, -8.2333, 8.3333) bodies 21 in component "Holey Cube"
mirror "Mirror3'" about plane through (25, -25, 0) normal (0, -1, 0) of 4 faces at (40.4068, -11.7889, 11.7983) (57.0735, -11.7889, 11.7983) (60.5982, -12.0056, 5.6186) (40.0306, -12.0056, 11.3404) on bodies 20 21 22 in component "Holey Cube"
mirror "Mirror4'" about plane through (100.3, -50, 12.7) normal (1, 0, 0) of bodies 23 22 24 20 21 makes body 25 at (188.1, -29.1673, 42.9228) makes body 26 at (129.5178, -42.9153, 12.5) makes body 27 at (147.7217, -20.9, 0) makes body 28 at (100.3, -38.8889, 20.9) makes body 29 at (179.7, 0.1, 44.4444) in component "Holey Cube"
combine "Combine2'" operation add target body 23 tool bodies 28 in component "Holey Cube"
mirror "Mirror5'" about plane through (187.9, 0.1, 50) normal (0, 1, 0) of bodies 29 23 21 27 20 24 26 22 25 makes body 30 at (12.5, 29.3673, 42.9228) makes body 31 at (71.0822, 43.1153, 12.5) makes body 32 at (52.8783, 21.1, 0) makes body 33 at (97.5217, 50.2, 29.1) makes body 34 at (20.9, 0.1, 38.8889) makes body 35 at (188.1, 29.3673, 42.9228) makes body 36 at (129.5178, 43.1153, 12.5) makes body 37 at (147.7217, 29.3, 0) makes body 38 at (179.7, 0.1, 44.4444) in component "Holey Cube"
combine "Combine3'" operation add target body 24 tool bodies 34 in component "Holey Cube"
combine "Combine4'" operation add target body 29 tool bodies 38 in component "Holey Cube"
move_body "Move1" bodies 32 25 21 36 27 30 35 37 26 20 23 29 24 31 33 22 to x (1, 0, 0) y (0, 1, 0) z (0, 0, 1) at (-250, 0, 0) in component "Holey Cube"
sketch "Sketch1 (3)" plane through (0, 0, 0) normal (0, 0, 1) x (1, 0, 0) in component "Cube HalfSpace"
  line L0 (0, 0) -> (25, 0)
  line L1 (25, 0) -> (25, -25)
  line L2 (25, -25) -> (0, -25)
  line L3 (0, -25) -> (0, 0)
  line L4 (25.1, 0) -> (50.1, 0)
  line L5 (50.1, 0) -> (50.1, -25)
  line L6 (50.1, -25) -> (25.1, -25)
  line L7 (25.1, -25) -> (25.1, 0)
  dimension "d1_1" = 50
  dimension "d2_1" = 50
  dimension "d3_1" = 50
  dimension "d4_1" = 50
  dimension "d5_1" = 0.1
  constraint horizontal L0
  constraint vertical L1
  constraint horizontal L2
  constraint vertical L3
  constraint coincident L0.start L3.end
  constraint horizontal L4
  constraint vertical L5
  constraint horizontal L6
  constraint vertical L7
  constraint collinear L0 L4
  measures "d5_1" distance of L1 L7
extrude "Extrude1''" [suppressed] in component "Cube HalfSpace"
sketch "Sketch2 (3)" plane through (0, 0, 0) normal (0, 0, -1) x (1, 0, 0) in component "Cube HalfSpace"
  line L0 (25, 25) -> (0, 25)
  line L1 (0, 25) -> (0, 0)
  line L2 (0, 0) -> (25, 0)
  line L3 (25, 0) -> (25, 25)
  line L4 (25, 6.5) -> (14.9, 6.5)
  line L5 (14.9, 6.5) -> (14.9, 18.5)
  line L6 (14.9, 18.5) -> (25, 18.5)
  line L7 (25, 18.5) -> (25, 6.5)
  line L8 (25.05, 6.6) -> (15, 6.6)
  line L9 (15, 6.6) -> (15, 18.4)
  line L10 (15, 18.4) -> (25.05, 18.4)
  line L11 (25.05, 18.4) -> (25.05, 6.6)
  line L12 (0, 12.5) -> (25, 12.5) construction
  dimension "d8_1" = 0.05
  dimension "d9_1" = 0.1
  dimension "d10_1" = 0.1
  dimension "d11_1" = 0.1
  dimension "d12_1" = 25
  dimension "d13_1" = 16.7667
  constraint horizontal L4
  constraint vertical L5
  constraint horizontal L6
  constraint vertical L7
  constraint coincident L3 L4.start
  constraint horizontal L8
  constraint vertical L9
  constraint horizontal L10
  constraint vertical L11
  constraint midpoint L1 L12.start
  constraint midpoint L3 L12.end
  constraint symmetric L4 L6 L12
  measures "d8_1" distance of L7 L11
  measures "d9_1" distance of L4 L8
  measures "d10_1" distance of L6 L10
  measures "d11_1" distance of L5 L9
sketch "Sketch3 (3)" plane through (0, 0, 0) normal (0, 0, -1) x (1, 0, 0) in component "Cube HalfSpace"
  line L0 (50.1, 25) -> (25.1, 25)
  line L1 (25.1, 25) -> (25.1, 0)
  line L2 (25.1, 0) -> (50.1, 0)
  line L3 (50.1, 0) -> (50.1, 25)
  line L4 (50.1, 12.5) -> (25.1, 12.5) construction
  line L5 (35.2, 6.5) -> (25.1, 6.5)
  line L6 (25.1, 6.5) -> (25.1, 18.5)
  line L7 (25.1, 18.5) -> (35.2, 18.5)
  line L8 (35.2, 18.5) -> (35.2, 6.5)
  line L9 (35.1, 6.6) -> (25.05, 6.6)
  line L10 (25.05, 6.6) -> (25.05, 18.4)
  line L11 (25.05, 18.4) -> (35.1, 18.4)
  line L12 (35.1, 18.4) -> (35.1, 6.6)
  dimension "d19_1" = 0.1
  dimension "d20_1" = 0.1
  dimension "d21_1" = 0.1
  dimension "d22_1" = 25
  dimension "d23_1" = 0.05
  dimension "d24_1" = 16.7667
  constraint midpoint L3 L4.start
  constraint midpoint L1 L4.end
  constraint horizontal L5
  constraint vertical L6
  constraint horizontal L7
  constraint vertical L8
  constraint coincident L1 L6.end
  constraint horizontal L9
  constraint vertical L10
  constraint horizontal L11
  constraint vertical L12
  constraint symmetric L4 L5 L7
  measures "d19_1" distance of L5 L9
  measures "d20_1" distance of L8 L12
  measures "d21_1" distance of L7 L11
  measures "d23_1" distance of L6 L10
sketch "Sketch4 (3)" plane through (0, 0, 20) normal (0, 0, 1) x (-1, 0, 0) in component "Cube HalfSpace"
  line L0 (0, 25) -> (-25, 25)
  line L1 (-25, 25) -> (-25, 0)
  line L2 (-25, 0) -> (0, 0)
  line L3 (0, 0) -> (0, 25)
  line L4 (-12.5, 25) -> (-12.5, 0) construction
  line L5 (-18.5, 10.1) -> (-6.5, 10.1)
  line L6 (-6.5, 10.1) -> (-6.5, 0)
  line L7 (-6.5, 0) -> (-18.5, 0)
  line L8 (-18.5, 0) -> (-18.5, 10.1)
  line L9 (-18.4, 10) -> (-6.6, 10)
  line L10 (-6.6, 10) -> (-6.6, -0.05)
  line L11 (-6.6, -0.05) -> (-18.4, -0.05)
  line L12 (-18.4, -0.05) -> (-18.4, 10)
  dimension "d25_1" = 0.05
  dimension "d26_1" = 0.1
  dimension "d27_1" = 0.1
  dimension "d28_1" = 25
  dimension "d29_1" = 0.1
  dimension "d30_1" = 16.7667
  constraint midpoint L0 L4.start
  constraint midpoint L2 L4.end
  constraint horizontal L5
  constraint vertical L6
  constraint horizontal L7
  constraint vertical L8
  constraint coincident L2 L6.end
  constraint horizontal L9
  constraint vertical L10
  constraint horizontal L11
  constraint vertical L12
  measures "d25_1" distance of L7 L11
  measures "d26_1" distance of L8 L12
  measures "d27_1" distance of L6 L10
  measures "d29_1" distance of L5 L9
sketch "Sketch5 (3)" plane through (0, 0, 20) normal (0, 0, 1) x (-1, 0, 0) in component "Cube HalfSpace"
  line L0 (-25.1, 25) -> (-50.1, 25)
  line L1 (-50.1, 25) -> (-50.1, 0)
  line L2 (-50.1, 0) -> (-25.1, 0)
  line L3 (-25.1, 0) -> (-25.1, 25)
  line L4 (-50.1, 12.5) -> (-25.1, 12.5) construction
  line L5 (-50.1, 18.5) -> (-40, 18.5)
  line L6 (-40, 18.5) -> (-40, 6.5)
  line L7 (-40, 6.5) -> (-50.1, 6.5)
  line L8 (-50.1, 6.5) -> (-50.1, 18.5)
  line L9 (-50.15, 18.4) -> (-40.1, 18.4)
  line L10 (-40.1, 18.4) -> (-40.1, 6.6)
  line L11 (-40.1, 6.6) -> (-50.15, 6.6)
  line L12 (-50.15, 6.6) -> (-50.15, 18.4)
  dimension "d31_1" = 0.05
  dimension "d32_1" = 0.1
  dimension "d33_1" = 0.1
  dimension "d34_1" = 0.1
  dimension "d35_1" = 16.7667
  dimension "d36_1" = 25
  constraint midpoint L1 L4.start
  constraint midpoint L3 L4.end
  constraint horizontal L5
  constraint vertical L6
  constraint horizontal L7
  constraint vertical L8
  constraint coincident L1 L5.start
  constraint horizontal L9
  constraint vertical L10
  constraint horizontal L11
  constraint vertical L12
  constraint symmetric L4 L5 L7
  measures "d31_1" distance of L8 L12
  measures "d32_1" distance of L7 L11
  measures "d33_1" distance of L5 L9
  measures "d34_1" distance of L6 L10
chamfer "Chamfer1''" [suppressed] in component "Cube HalfSpace"
extrude "Extrude2''" [suppressed] in component "Cube HalfSpace"